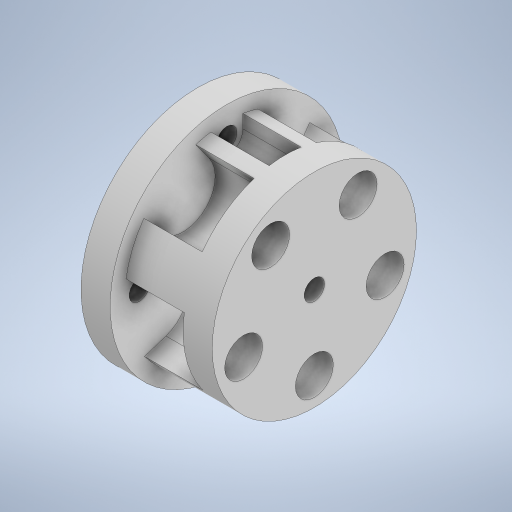
# Autodesk Inventor part: EaglePowerCycDriveAdaptor
Saved by Autodesk Inventor 2023 (Build 270158000, 158)
## iProperties
Created: 2023-03-29
Part Number: EaglePowerCycDriveAdaptor
Material: Generic
Document SubType Name: Sheet Metal
Designer: Charles Kelly
Density: 1 g/cm^3
Sheet Metal Rule: Default_mm
Appearance: Default
Author: Charles Kelly
Autodesk Inventor part; units mm, degrees
ref_plane "YZ Plane" through (0, 0, 0) normal (1, 0, 0) x (0, 1, 0)
ref_plane "XZ Plane" through (0, 0, 0) normal (0, 1, 0) x (-1, 0, 0)
ref_plane "XY Plane" through (0, 0, 0) normal (0, 0, 1) x (1, 0, 0)
sketch "Sketch1" plane through (0, 0, 0) normal (1, 0, 0) x (0, 1, 0)
  circle A0 centre (0, 0) radius 15
  circle A1 centre (15, 0) radius 1.75
  circle A2 centre (0, 15) radius 1.75
  circle A3 centre (-15, 0) radius 1.75
  circle A4 centre (0, -15) radius 1.75
  circle A5 centre (0, 0) radius 1.75
  circle A6 centre (0, 0) radius 20
  dimension "d0" = 30
  dimension "d1" = 3.5
  dimension "d4" = 360
  dimension "d6" = 3.5
  dimension "d7" = 40
  constraints: 6 centre point, 3 coincident, 1 horizontal alignment, 11 other
  measures "d1" diameter of A1
  measures "d6" diameter of A5
  measures "d7" diameter of A6
extrude "Extrusion1" add sketch "Sketch1" along normal blind 5 contours A1 A0 A4 A3 A2 | A6
sketch "Sketch2" plane through (5, 0, 0) normal (1, 0, 0) x (0, 0, -1)
  circle A0 centre (0, 0) radius 1.75
  circle A1 centre (0, 0) radius 12.75
  circle A2 centre (0, -12.75) radius 3.25
  circle A3 centre (12.126, -3.94) radius 3.25
  circle A4 centre (7.4943, 10.315) radius 3.25
  circle A5 centre (-7.4943, 10.315) radius 3.25
  circle A6 centre (-12.126, -3.94) radius 3.25
  circle A7 centre (0, 0) radius 1.75 projected
  circle A8 centre (0, 0) radius 17.5
  dimension "d10" = 25.5
  dimension "d11" = 6.5
  dimension "d14" = 360
  dimension "d16" = 35
  constraints: 7 centre point, 3 coincident, 1 vertical alignment, 13 other
  measures "d11" diameter of A2
  measures "d16" diameter of A8
extrude "Extrusion2" add sketch "Sketch2" along normal blind 15 contours A1 A3 A2 A6 A5 A4 | A8
sketch "Sketch3" plane through (5, 0, 0) normal (1, 0, 0) x (0, 0, -1)
  circle A0 centre (0, -12.75) radius 5.5
  line L0 (0, -12.75) -> (5.5, -12.75)
  line L1 (0, -12.75) -> (-5.5, -12.75)
  circle A1 centre (0, 0) radius 17.5 projected
  line L2 (-5.5, -16.6132) -> (-5.5, -12.75)
  line L3 (5.5, -16.6132) -> (5.5, -12.75)
  circle A2 centre (0, 0) radius 1.75 projected
  circle A3 centre (0, 0) radius 17.5
  line L4 (12.126, -3.94) -> (13.8256, 1.2908)
  line L5 (12.126, -3.94) -> (10.4264, -9.1708)
  circle A4 centre (12.126, -3.94) radius 5.5
  line L6 (17.4997, 0.097) -> (13.8256, 1.2908)
  line L7 (14.1005, -10.3646) -> (10.4264, -9.1708)
  line L8 (7.4943, 10.315) -> (3.0447, 13.5478)
  line L9 (7.4943, 10.315) -> (11.9439, 7.0821)
  circle A5 centre (7.4943, 10.315) radius 5.5
  line L10 (5.3154, 16.6732) -> (3.0447, 13.5478)
  line L11 (14.2146, 10.2076) -> (11.9439, 7.0821)
  line L12 (-7.4943, 10.315) -> (-11.9439, 7.0821)
  line L13 (-7.4943, 10.315) -> (-3.0447, 13.5478)
  circle A6 centre (-7.4943, 10.315) radius 5.5
  line L14 (-14.2146, 10.2076) -> (-11.9439, 7.0821)
  line L15 (-5.3154, 16.6732) -> (-3.0447, 13.5478)
  line L16 (-12.126, -3.94) -> (-10.4264, -9.1708)
  line L17 (-12.126, -3.94) -> (-13.8256, 1.2908)
  circle A7 centre (-12.126, -3.94) radius 5.5
  line L18 (-14.1005, -10.3646) -> (-10.4264, -9.1708)
  line L19 (-17.4997, 0.097) -> (-13.8256, 1.2908)
  point P0 (-12.126, -3.94)
  point P1 (15.3573, -8.3906)
  point P2 (17.3562, -2.2387)
  point P3 (-7.4925, 15.815)
  point P4 (-12.7256, 12.0128)
  point P5 (-17.3562, -2.2387)
  point P6 (-15.3573, -8.3906)
  dimension "d19" = 11
  dimension "d22" = 360
  constraints: 40 end point, 20 point on circle, 6 coincident, 5 centre point, 1 parallel, 1 perpendicular, 71 other
  measures "d19" diameter of A0
extrude "Extrusion3" cut sketch "Sketch3" along normal blind 10 contours L0 L1 A0 | L3 A1 A0 | A0 A1 L1 L0 | A0 A1 L2 | L7 A4 A1 | A1 A7 L18 | A4 L5 L4 A1 | A1 A4 | A4 L4 L5 | A7 A1 | A1 A7 L17 L16 | L16 L17 A7 | A4 L6 A1 | A1 L19 A7 | L11 A5 A1 | A1 A6 L14 | A5 L9 L8 A1 | A5 L8 L9 | A6 A1 | A1 A6 L13 L12 | L12 L13 A6 | A5 L10 A1 | A1 L15 A6
sketch "Sketch4" plane through (5, 0, 0) normal (1, 0, 0) x (0, 0, -1)
  circle A0 centre (0, -15) radius 1.75 projected
  circle A1 centre (0, -15) radius 2.75
  circle A2 centre (15, 0) radius 2.75
  circle A3 centre (0, 15) radius 2.75
  circle A4 centre (-15, 0) radius 2.75
  circle A5 centre (0, 0) radius 1.75 projected
  circle A6 centre (0, 0) radius 17.75
  line L0 (-2.75, -15) -> (-2.75, -17.5357)
  line L1 (2.75, -15) -> (2.75, -17.5357)
  line L2 (15, -2.75) -> (17.5357, -2.75)
  line L3 (15, 2.75) -> (17.5357, 2.75)
  line L4 (2.75, 15) -> (2.75, 17.5357)
  line L5 (-2.75, 15) -> (-2.75, 17.5357)
  line L6 (-15, 2.75) -> (-17.5357, 2.75)
  line L7 (-15, -2.75) -> (-17.5357, -2.75)
  point P0 (2.75, 15)
  dimension "d31" = 35.5
  dimension "d26" = 5.5
  dimension "d29" = 360
  dimension "d34" = 360
  constraints: 16 end point, 4 centre point, 2 coincident, 2 point on circle, 1 parallel, 1 vertical, 37 other
  measures "d26" diameter of A1
extrude "Extrusion4" cut sketch "Sketch4" along normal blind 10 contours A0 | A1 | L1 A6 A1 | A1 A6 L0 | L2 A2 A6 | A6 A4 L7 | A2 | A2 L3 A6 | A6 L6 A4 | A4 | L4 A3 A6 | A6 A3 L5 | A3 | A5
equation "\"BendRadius\" = Thickness"
equation "\"BendReliefWidth\" = Thickness"
equation "\"BendReliefDepth\" = 0.5 * Thickness"
equation "\"CornerReliefSize\" = 4 * Thickness"
equation "\"MinimumRemnant\" = 2 * Thickness"
equation "\"TransitionRadius\" = BendRadius"
equation "\"JacobiRadiusSize\" = BendRadius"
equation "\"GapSize\" = Thickness"
equation "\"Thickness\" = 0.5"
body "Solid1"
